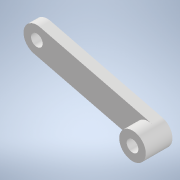
# Autodesk Inventor part: union_yema
Saved by Autodesk Inventor 2020 (Build 240168000, 168)
## iProperties
Created: 2021-08-05
Part Number: union_yema
Material: PC/ABS Plastic
Document SubType Name: Modeling
Designer: chalo
Density: 0.357273 g/cm^3
Appearance: Smooth - White
Author: chalo
Autodesk Inventor part; units mm, degrees
ref_plane "YZ Plane" through (0, 0, 0) normal (1, 0, 0) x (0, 1, 0)
sketch "Sketch1" plane through (0, 0, 0) normal (0, 0, 1) x (1, 0, 0)
  circle A0 centre (6.2788, 3.6472) radius 1.1 projected
  arc A1 (5.219, 1.9512) -> (4.2801, 3.717) centre (6.2788, 3.6472) ccw projected
  line L0 (4.2801, 3.717) -> (-5.6503, -1.563) projected
  line L1 (-7.3788, -4.7472) -> (-5.6503, -1.563) projected
  line L2 (-7.3788, -4.7472) -> (5.219, 1.9512) projected
  circle A2 centre (6.2788, 3.6472) radius 2.5
  circle A3 centre (27.2459, -1.5472) radius 1.1 projected
  circle A4 centre (27.2459, -1.5472) radius 2.5
  line L3 (5.6777, 1.2206) -> (26.6447, -3.9739)
  line L4 (6.88, 6.0739) -> (27.8471, 0.8794)
  point P0 (0, 0)
  dimension "d0" = 5
  dimension "d1" = 5
  constraints: 4 end point, 4 point on circle, 4 tangent, 2 centre point, 2 coincident
  measures "d0" diameter of A2
  measures "d1" diameter of A4
extrude "Extrusion1" add sketch "Sketch1" along normal blind 2 contours L2 A2 L0 A1 | A1 L0 A2 L2 | A2 L4 A4 L3 | A4
sketch "Sketch2" plane through (0, 0, 2) normal (0, 0, 1) x (1, 0, 0)
  arc A0 (26.6447, -3.9739) -> (27.8471, 0.8794) centre (27.2459, -1.5472) ccw projected
  line L0 (27.8471, 0.8794) -> (6.88, 6.0739) projected
  arc A1 (6.88, 6.0739) -> (5.6777, 1.2206) centre (6.2788, 3.6472) ccw projected
  line L1 (5.6777, 1.2206) -> (26.6447, -3.9739) projected
  circle A2 centre (27.2459, -1.5472) radius 1.1 projected
  circle A3 centre (6.2788, 3.6472) radius 1.1 projected
  arc A4 (26.6447, -3.9739) -> (27.8471, 0.8794) centre (27.2459, -1.5472) ccw projected
  circle A5 centre (27.2459, -1.5472) radius 2.5
  point P0 (0, 0)
  point P1 (27.8471, 0.8794)
  point P2 (26.6447, -3.9739)
  dimension "d4" = 5
  constraints: 1 centre point, 1 coincident
  measures "d4" diameter of A5
ref_plane "Work Plane1" through (24.6322, -7.0775, 5) normal (0, 0, 1) x (1, 0, 0)
ref_plane "Work Plane2" through (24.6969, -3.0472, 3) normal (0, 0, -1) x (0, 1, 0)
extrude "Extrusion2" add sketch "Sketch2" along normal up to surface (1 mm away) contours A5 A0
body "Solid1"
